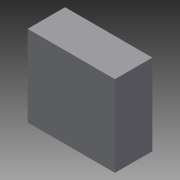
# Autodesk Inventor part: Battery
Saved by Autodesk Inventor 2013 (Build 170138000, 138)
## iProperties
Created: 2014-01-31
Part Number: Battery
Material: Generic
Document SubType Name: Modeling
Designer: 215152
Density: 1 g/cm^3
Author: 215152
Autodesk Inventor part; units mm, degrees
ref_plane "YZ Plane" through (0, 0, 0) normal (1, 0, 0) x (0, 1, 0)
ref_plane "XZ Plane" through (0, 0, 0) normal (0, 1, 0) x (-1, 0, 0)
ref_plane "XY Plane" through (0, 0, 0) normal (0, 0, 1) x (1, 0, 0)
sketch "Sketch1" plane through (0, 0, 0) normal (0, 1, 0) x (-1, 0, 0)
  line L0 (-88.9, -38.1) -> (88.9, -38.1)
  line L1 (88.9, -38.1) -> (88.9, 38.1)
  line L2 (88.9, 38.1) -> (-88.9, 38.1)
  line L3 (-88.9, 38.1) -> (-88.9, -38.1)
  line L4 (-88.9, -38.1) -> (88.9, 38.1) construction
  line L5 (88.9, -38.1) -> (-88.9, 38.1) construction
  point P0 (0, 0)
  dimension "d0" = 177.8
  dimension "d1" = 76.2
  constraints: 12 end point, 2 midpoint, 2 parallel, 1 horizontal, 1 perpendicular
  measures "d0" distance of L2.end L1.end
  measures "d1" distance of L1.end L0.end
extrude "Extrusion1" add sketch "Sketch1" along normal blind 165.1
body "Solid1"
